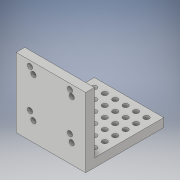
# Autodesk Inventor part: LidarMount2
Saved by Autodesk Inventor 2019 (Build 230136000, 136)
## iProperties
Created: 2020-03-02
Part Number: LidarMount2
Material: Generic
Document SubType Name: Modeling
Designer: james
Density: 1 g/cm^3
Appearance: Default
Author: james
Autodesk Inventor part; units mm, degrees
ref_plane "YZ Plane" through (0, 0, 0) normal (1, 0, 0) x (0, 1, 0)
ref_plane "XZ Plane" through (0, 0, 0) normal (0, 1, 0) x (-1, 0, 0)
ref_plane "XY Plane" through (0, 0, 0) normal (0, 0, 1) x (1, 0, 0)
sketch "Sketch1" plane through (0, 0, 0) normal (0, 0, 1) x (1, 0, 0)
  line L0 (-31.4222, 23.2631) -> (19.3778, 23.2631)
  line L1 (19.3778, 23.2631) -> (19.3778, -21.1869)
  line L2 (19.3778, -21.1869) -> (-31.4222, -21.1869)
  line L3 (-31.4222, -21.1869) -> (-31.4222, 23.2631)
  point P0 (0, 0)
  dimension "d0" = 44.45
  dimension "d1" = 50.8
  constraints: 8 end point, 2 parallel, 1 horizontal, 1 perpendicular
  measures "d0" distance of L2.end L0.start
  measures "d1" distance of L0.start L0.end
extrude "Extrusion1" add sketch "Sketch1" along normal blind 6.35
sketch "Sketch2" plane through (0, 0, 6.35) normal (0, 0, 1) x (1, 0, 0)
  line L0 (-31.4222, -21.1869) -> (19.3778, -21.1869)
  line L1 (19.3778, -21.1869) -> (19.3778, -27.5369)
  line L2 (19.3778, -27.5369) -> (-31.4222, -27.5369)
  line L3 (-31.4222, -27.5369) -> (-31.4222, -21.1869)
  line L4 (19.3778, -21.1869) -> (19.3778, 23.2631) projected
  line L5 (-31.4222, 23.2631) -> (-31.4222, -21.1869) projected
  line L6 (-31.4222, -21.1869) -> (19.3778, -21.1869) projected
  point P0 (0, 0)
  dimension "d4" = 0
  dimension "d5" = 0
  dimension "d6" = 6.35
  dimension "d7" = 0
  constraints: 8 end point, 2 parallel, 1 horizontal, 1 perpendicular
  measures "d4" distance between parallel lines of L4 L1
  measures "d5" distance between parallel lines of L5 L3
  measures "d6" distance between parallel lines of L0 L2
  measures "d7" distance between parallel lines of L6 L0
extrude "Extrusion2" add sketch "Sketch2" against normal blind 57.15
sketch "Sketch3" plane through (0, 0, 6.35) normal (0, 0, 1) x (1, 0, 0)
  line L0 (19.3778, 23.2631) -> (-31.4222, 23.2631) projected
  line L1 (-31.4222, 23.2631) -> (-31.4222, -27.5369) projected
  line L2 (19.3778, 23.2631) -> (19.3778, -27.5369) projected
  point P0 (0, 0)
  point P1 (-21.2622, 19.4531)
  point P2 (-21.2622, -8.4869)
  point P3 (7.9478, 19.4531)
  point P4 (7.9478, -8.4869)
  dimension "d10" = 29.21
  dimension "d11" = 0
  dimension "d12" = 0
  dimension "d13" = 0
  dimension "d14" = 27.94
  dimension "d15" = 3.81
  dimension "d16" = 10.16
  dimension "d17" = 11.43
  dimension "d25" = 0
  measures "d10" distance of point (7.948, -8.487) point (-21.262, -8.487)
  measures "d11" horizontal distance of point (-21.262, -8.487) point (-21.262, 19.453)
  measures "d12" horizontal distance of point (7.948, -8.487) point (7.948, 19.453)
  measures "d13" vertical distance of point (-21.262, 19.453) point (7.948, 19.453)
  measures "d14" distance of point (-21.262, -8.487) point (-21.262, 19.453)
  measures "d15" distance from line of L0 point (-21.262, 19.453)
  measures "d16" distance from line of L1 point (-21.262, 19.453)
  measures "d17" distance from line of L2 point (7.948, 19.453)
  measures "d25" vertical distance of point (-21.262, -8.487) point (7.948, -8.487)
hole "Hole1" at (-21.2622, 19.4531, 6.35) at (-21.2622, -8.4869, 6.35) at (7.9478, 19.4531, 6.35) at (7.9478, -8.4869, 6.35) direction (0, 0, -1) diameter 3.81 depth 25.4 tip angle 118
sketch "Sketch4" plane through (0, 0, 6.35) normal (0, 0, 1) x (1, 0, 0)
  circle A0 centre (-21.2622, 19.4531) radius 1.905 projected
  point P0 (0, 0)
  point P1 (-18.7222, 15.6431)
  point P2 (9.2178, 15.6431)
  point P3 (9.2178, -13.5669)
  point P4 (-18.7222, -13.5669)
  dimension "d26" = 0
  dimension "d27" = 0
  dimension "d28" = 0
  dimension "d29" = 0
  dimension "d30" = 29.21
  dimension "d31" = 27.94
  dimension "d42" = 2.54
  dimension "d43" = 3.81
  measures "d26" horizontal distance of point (-18.722, -13.567) point (-18.722, 15.643)
  measures "d27" horizontal distance of point (9.218, -13.567) point (9.218, 15.643)
  measures "d28" vertical distance of point (-18.722, 15.643) point (9.218, 15.643)
  measures "d29" vertical distance of point (-18.722, -13.567) point (9.218, -13.567)
  measures "d30" distance of point (-18.722, -13.567) point (-18.722, 15.643)
  measures "d31" distance of point (9.218, 15.643) point (-18.722, 15.643)
  measures "d42" horizontal distance of A0.centre point (-18.722, 15.643)
  measures "d43" vertical distance of A0.centre point (-18.722, 15.643)
hole "Hole2" at (-18.7222, 15.6431, 6.35) at (9.2178, 15.6431, 6.35) at (9.2178, -13.5669, 6.35) at (-18.7222, -13.5669, 6.35) direction (0, 0, -1) diameter 3.81 depth 25.4 tip angle 118
sketch "Sketch5" plane through (-31.4222, -21.1869, 0) normal (0, 1, 0) x (1, 0, 0)
  line L0 (50.8, 0) -> (50.8, 50.8) projected
  line L1 (0, 50.8) -> (50.8, 50.8) projected
  point P0 (31.4222, 0)
  point P1 (44.45, 44.45)
  point P2 (44.45, 36.83)
  point P3 (44.45, 29.21)
  point P4 (44.45, 21.59)
  point P5 (44.45, 13.97)
  point P6 (44.45, 6.35)
  point P7 (36.83, 6.35)
  point P8 (36.83, 13.97)
  point P9 (36.83, 21.59)
  point P10 (36.83, 29.21)
  point P11 (36.83, 36.83)
  point P12 (36.83, 44.45)
  point P13 (29.21, 6.35)
  point P14 (29.21, 13.97)
  point P15 (29.21, 21.59)
  point P16 (29.21, 29.21)
  point P17 (29.21, 36.83)
  point P18 (29.21, 44.45)
  point P19 (21.59, 6.35)
  point P20 (21.59, 13.97)
  point P21 (21.59, 21.59)
  point P22 (21.59, 29.21)
  point P23 (21.59, 36.83)
  point P24 (21.59, 44.45)
  point P25 (13.97, 6.35)
  point P26 (13.97, 13.97)
  point P27 (13.97, 21.59)
  point P28 (13.97, 29.21)
  point P29 (13.97, 36.83)
  point P30 (13.97, 44.45)
  point P31 (6.35, 6.35)
  point P32 (6.35, 13.97)
  point P33 (6.35, 21.59)
  point P34 (6.35, 29.21)
  point P35 (6.35, 36.83)
  point P36 (6.35, 44.45)
  dimension "d44" = 6.35
  dimension "d45" = 6.35
  dimension "d48" = 7.62
  dimension "d58" = 7.62
  constraints: 1 horizontal, 1 vertical, 35 other
  measures "d44" distance from line of L0 point (44.45, 44.45)
  measures "d45" distance from line of L1 point (44.45, 44.45)
  measures "d48" distance of point (44.45, 44.45) point (44.45, 36.83)
  measures "d58" distance of point (44.45, 6.35) point (36.83, 6.35)
hole "Hole3" at (13.0278, -21.1869, -44.45) at (13.0278, -21.1869, -36.83) at (13.0278, -21.1869, -29.21) at (13.0278, -21.1869, -21.59) at (13.0278, -21.1869, -13.97) at (13.0278, -21.1869, -6.35) at (5.4078, -21.1869, -6.35) at (5.4078, -21.1869, -13.97) at (5.4078, -21.1869, -21.59) at (5.4078, -21.1869, -29.21) at (5.4078, -21.1869, -36.83) at (5.4078, -21.1869, -44.45) at (-2.2122, -21.1869, -6.35) at (-2.2122, -21.1869, -13.97) at (-2.2122, -21.1869, -21.59) at (-2.2122, -21.1869, -29.21) at (-2.2122, -21.1869, -36.83) at (-2.2122, -21.1869, -44.45) at (-9.8322, -21.1869, -6.35) at (-9.8322, -21.1869, -13.97) at (-9.8322, -21.1869, -21.59) at (-9.8322, -21.1869, -29.21) at (-9.8322, -21.1869, -36.83) at (-9.8322, -21.1869, -44.45) at (-17.4522, -21.1869, -6.35) at (-17.4522, -21.1869, -13.97) at (-17.4522, -21.1869, -21.59) at (-17.4522, -21.1869, -29.21) at (-17.4522, -21.1869, -36.83) at (-17.4522, -21.1869, -44.45) at (-25.0722, -21.1869, -6.35) at (-25.0722, -21.1869, -13.97) at (-25.0722, -21.1869, -21.59) at (-25.0722, -21.1869, -29.21) at (-25.0722, -21.1869, -36.83) at (-25.0722, -21.1869, -44.45) direction (0, -1, 0) diameter 3.81 depth 25.4 tip angle 118
body "Solid1"
